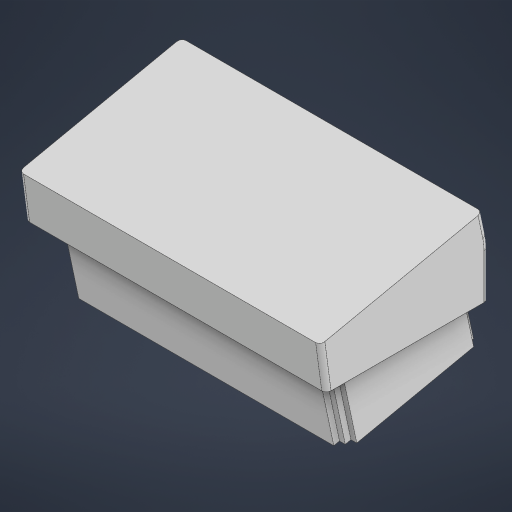
# Autodesk Inventor part: outer
Saved by Autodesk Inventor 2024.2 (Build 282272000, 272)
## iProperties
Created: 2024-08-19
Part Number: outer
Material: Generic
Document SubType Name: Modeling
Designer: Moe
Density: 1 g/cm^3
Appearance: Default
Author: Moe
Autodesk Inventor part; units mm, degrees
ref_plane "YZ Plane" through (0, 0, 0) normal (1, 0, 0) x (0, 1, 0)
ref_plane "XZ Plane" through (0, 0, 0) normal (0, 1, 0) x (-1, 0, 0)
ref_plane "XY Plane" through (0, 0, 0) normal (0, 0, 1) x (1, 0, 0)
sketch "Sketch1" plane through (0, 0, 0) normal (1, 0, 0) x (0, 1, 0)
  line L0 (0, 0) -> (0, -70)
  line L1 (0, 0) -> (70, 0) construction
  line L2 (0, 0) -> (7, 0)
  line L3 (7, 0) -> (21.879, -70)
  line L4 (7, 0) -> (78.5638, 0) construction
  line L5 (21.879, -70) -> (0, -70)
  dimension "d0" = 70
  dimension "d1" = 90
  dimension "d2" = 7
  dimension "d3" = 78
  constraints: 12 end point, 3 horizontal, 2 equal length, 1 point on line, 1 vertical
  measures "d0" distance of L0.start L0.end
  measures "d1" angle of L0 L1
  measures "d2" distance of L0.start L2.end
  measures "d3" angle of L3 L4
extrude "Extrusion1" add sketch "Sketch1" along normal blind 130
sketch "Sketch2" plane through (0, 7, 0) normal (0, 0.9781476, 0.2079117) x (1, 0, 0)
  line L0 (5, 64.9998) -> (125, 64.9998)
  line L1 (125, 64.9998) -> (125, 5)
  line L2 (125, 5) -> (5, 5)
  line L3 (5, 5) -> (5, 64.9998)
  line L4 (0, 71.5638) -> (130, 71.5638) projected
  line L5 (0, 71.5638) -> (0, 0) projected
  line L6 (0, 0) -> (130, 0) projected
  line L7 (130, 71.5638) -> (130, 0) projected
  point P0 (0, -1.4554)
  dimension "d6" = 6.564
  dimension "d7" = 5
  dimension "d8" = 5
  dimension "d9" = 5
  dimension "d71" = 59.9998
  dimension "d72" = 120
  constraints: 8 end point, 2 parallel, 1 horizontal, 1 perpendicular
  measures "d6" distance between parallel lines of L4 L0
  measures "d7" distance between parallel lines of L5 L3
  measures "d8" distance between parallel lines of L6 L2
  measures "d9" distance between parallel lines of L7 L1
  measures "d71" distance of L2.end L0.start
  measures "d72" distance of L1.end L2.end
ref_plane "Work Plane1" through (0, 25, -70) normal (0, -1, 0) x (1, 0, 0)
sketch "Sketch3" plane through (0, 25, -70) normal (0, -1, 0) x (1, 0, 0)
  line L0 (5, 65.1093) -> (5, 6.4206) projected
  line L1 (5, 6.4206) -> (125, 6.4206) projected
  line L2 (125, 65.1093) -> (5, 65.1093) projected
  line L3 (125, 6.4206) -> (125, 65.1093) projected
  line L4 (10, 6.4206) -> (10, 11.4206)
  line L5 (10, 11.4206) -> (5, 11.4206)
  line L6 (5, 65.1093) -> (10, 65.1093)
  line L7 (10, 65.1093) -> (10, 60.1093)
  line L8 (10, 60.1093) -> (5, 60.1093)
  line L9 (5, 60.1093) -> (5, 65.1093)
  line L10 (125, 65.1093) -> (120, 65.1093)
  line L11 (120, 65.1093) -> (120, 60.1093)
  line L12 (120, 60.1093) -> (125, 60.1093)
  line L13 (125, 60.1093) -> (125, 65.1093)
  line L14 (125, 6.4206) -> (120, 6.4206)
  line L15 (120, 6.4206) -> (120, 11.4206)
  line L16 (120, 11.4206) -> (125, 11.4206)
  line L17 (125, 11.4206) -> (125, 6.4206)
  circle A0 centre (7.5, 8.9206) radius 1.1
  circle A1 centre (7.5, 62.6093) radius 1.1
  circle A2 centre (122.5, 62.6093) radius 1.1
  circle A3 centre (122.5, 7.3907) radius 1.1
  point P0 (0, 70)
  dimension "d13" = 5
  dimension "d14" = 5
  dimension "d15" = 5
  dimension "d16" = 5
  dimension "d17" = 5
  dimension "d18" = 5
  dimension "d19" = 5
  dimension "d20" = 5
  dimension "d21" = 2.2
  dimension "d22" = 2.5
  dimension "d23" = 2.5
  dimension "d24" = 2.2
  dimension "d25" = 2.2
  dimension "d26" = 2.2
  constraints: 28 end point, 6 parallel, 5 perpendicular, 4 centre point, 3 horizontal, 2 point on line
  measures "d13" distance of L4.end L5.end
  measures "d14" distance of L4.start L4.end
  measures "d15" distance of L7.end L8.end
  measures "d16" distance of L6.end L7.end
  measures "d17" distance of L12.end L11.end
  measures "d18" distance of L11.end L10.end
  measures "d19" distance of L15.end L16.end
  measures "d20" distance of L14.end L15.end
  measures "d21" diameter of A0
  measures "d22" distance from line of L1 A0.centre
  measures "d23" distance from line of L0 A0.centre
  measures "d24" diameter of A1
  measures "d25" diameter of A2
  measures "d26" diameter of A3
extrude "Extrusion2" cut sketch "Sketch3" along normal blind 22 contours L2 L7 L8 L0 | L8 L7 L2 L11 L12 L3 L16 L15 L1 L4 L5 L0 | L5 L4 L1 L0 | L2 L3 L12 L11 | L15 L16 L3 L1 A3 | A3 L1 | A0 | A1 | A2 picked at (122.1539, 7.5953)
sketch "Sketch4" plane through (0, 7, 0) normal (0, 0.9781476, 0.2079117) x (1, 0, 0)
  line L0 (125, 5) -> (5, 5) projected
  line L1 (5, 5) -> (10, 5)
  line L2 (10, 5) -> (10, 10)
  line L3 (10, 10) -> (5, 10)
  line L4 (5, 10) -> (5, 5)
  line L5 (125, 5) -> (125, 3.9522) projected
  line L6 (125, 5) -> (120, 5)
  line L7 (120, 5) -> (120, 10)
  line L8 (120, 10) -> (125, 10)
  line L9 (125, 10) -> (125, 5)
  line L10 (125, 66.5546) -> (120, 66.5546)
  line L11 (120, 66.5546) -> (120, 61.5546)
  line L12 (120, 61.5546) -> (125, 61.5546)
  line L13 (125, 61.5546) -> (125, 66.5546)
  line L14 (5, 66.5546) -> (10, 66.5546)
  line L15 (10, 66.5546) -> (10, 61.5546)
  line L16 (10, 61.5546) -> (5, 61.5546)
  line L17 (5, 61.5546) -> (5, 66.5546)
  point P0 (0, -1.4554)
  dimension "d27" = 5
  dimension "d28" = 5
  dimension "d29" = 5
  dimension "d30" = 5
  dimension "d31" = 5
  dimension "d32" = 5
  dimension "d33" = 5
  dimension "d34" = 5
  constraints: 32 end point, 8 parallel, 4 horizontal, 4 perpendicular, 1 point on line
  measures "d27" distance of L3.end L2.end
  measures "d28" distance of L2.end L1.end
  measures "d29" distance of L7.end L8.end
  measures "d30" distance of L6.end L7.end
  measures "d31" distance of L12.end L11.end
  measures "d32" distance of L11.end L10.end
  measures "d33" distance of L15.end L16.end
  measures "d34" distance of L14.end L15.end
extrude "Extrusion3" add sketch "Sketch4" against normal blind 8 contours L0 L7 L8 L9 | L0 L4 L3 L2
extrude "Extrusion4" add sketch "Sketch4" against normal blind 20 contours L13 L12 L11 L10 | L14 L15 L16 L17
sketch "Sketch5" plane through (0, 7, 0) normal (0, 0.9781476, 0.2079117) x (1, 0, 0)
  line L0 (5, 10) -> (5, 61.5546) projected
  line L1 (5, 61.5546) -> (10, 61.5546) projected
  line L2 (10, 61.5546) -> (10, 64.9998) projected
  line L3 (10, 64.9998) -> (120, 64.9998) projected
  line L4 (125, 61.5546) -> (125, 10) projected
  line L5 (120, 64.9998) -> (120, 61.5546) projected
  line L6 (120, 61.5546) -> (125, 61.5546) projected
  line L7 (125, 10) -> (120, 10) projected
  line L8 (120, 10) -> (120, 5) projected
  line L9 (125, 5) -> (120, 5) projected
  line L10 (120, 5) -> (10, 5) projected
  line L11 (10, 5) -> (5, 5) projected
  line L12 (10, 5) -> (10, 10) projected
  line L13 (10, 10) -> (5, 10) projected
  line L14 (0, 71.5638) -> (0, 0) projected
  line L15 (0, 0) -> (130, 0) projected
  line L16 (130, 71.5638) -> (130, 0) projected
  line L17 (0, 71.5638) -> (130, 71.5638) projected
  line L18 (7.5, 7.5) -> (122.5, 7.5)
  line L19 (122.5, 7.5) -> (122.5, 64.0546)
  line L20 (122.5, 64.0546) -> (7.5, 64.0546)
  line L21 (7.5, 64.0546) -> (7.5, 7.5)
  point P0 (0, -1.4554)
  point P1 (10, 64.0546)
  point P2 (120, 64.0546)
  point P3 (122.5, 61.5546)
  point P4 (122.5, 10)
  point P5 (7.5, 10)
  point P6 (7.5, 61.5546)
  point P7 (120, 7.5)
  point P8 (10, 7.5)
  constraints: 8 end point, 2 parallel, 1 horizontal, 1 perpendicular
extrude "Extrusion5" add sketch "Sketch5" against normal blind 40 contours L0 L1 L21 L13 | L21 L1 L2 L20 L5 L6 L19 L7 L8 L18 L12 L13 | L21 L20 L2 L1 | L18 L8 L10 L12 | L2 L3 L5 L20 | L8 L7 L19 L18 | L20 L19 L6 L5 | L19 L6 L4 L7
sketch "Sketch6" plane through (125, 0, -11.7113) normal (1, 0, 0) x (0, 0, -1)
  line L0 (-11.7113, 0) -> (76.9148, 0)
  line L1 (76.9148, 0) -> (76.9148, -64.0889)
  line L2 (76.9148, -64.0889) -> (-11.7113, -64.0889)
  line L3 (-11.7113, -64.0889) -> (-11.7113, 0)
  constraints: 8 end point, 2 parallel, 1 horizontal, 1 perpendicular
extrude "Extrusion6" [suppressed]
fillet "Fillet1" [suppressed]
extrude "Extrusion7" add sketch "Sketch2" along normal blind 5.1
extrude "Extrusion8" add sketch "Sketch4" along normal blind 5.1
sketch "Sketch7" plane through (0, 11.9886, 1.0603) normal (0, 0.9781476, 0.2079117) x (1, 0, 0)
  line L0 (130, 0) -> (130, 71.5638) projected
  line L1 (130, 71.5638) -> (0, 71.5638) projected
  line L2 (0, 71.5638) -> (0, 0) projected
  line L3 (0, 0) -> (130, 0) projected
  line L4 (10, 64.9998) -> (120, 64.9998) projected
  line L5 (125, 61.5546) -> (125, 10) projected
  line L6 (120, 64.9998) -> (120, 61.5546) projected
  line L7 (120, 61.5546) -> (125, 61.5546) projected
  line L8 (125, 10) -> (120, 10) projected
  line L9 (120, 10) -> (120, 5) projected
  line L10 (120, 5) -> (10, 5) projected
  line L11 (10, 5) -> (10, 10) projected
  line L12 (10, 10) -> (5, 10) projected
  line L13 (5, 10) -> (5, 61.5546) projected
  line L14 (5, 61.5546) -> (10, 61.5546) projected
  line L15 (10, 61.5546) -> (10, 64.9998) projected
  line L16 (5, 5) -> (5, 3.9522) projected
  line L17 (10, 10) -> (5, 10)
  line L18 (5, 10) -> (5, 5)
  line L19 (5, 5) -> (10, 5)
  line L20 (10, 5) -> (10, 10)
  line L21 (10, 61.5546) -> (5, 61.5546)
  line L22 (5, 61.5546) -> (5, 66.5546)
  line L23 (5, 66.5546) -> (10, 66.5546)
  line L24 (10, 66.5546) -> (10, 61.5546)
  line L25 (120, 61.5546) -> (125, 61.5546)
  line L26 (125, 61.5546) -> (125, 66.5546)
  line L27 (125, 66.5546) -> (120, 66.5546)
  line L28 (120, 66.5546) -> (120, 61.5546)
  line L29 (125, 10) -> (120, 10)
  line L30 (120, 10) -> (120, 5)
  line L31 (120, 5) -> (125, 5)
  line L32 (125, 5) -> (125, 10)
  point P0 (0, -1.4554)
  point P1 (5, 61.5546)
  point P2 (5, 61.5546)
  point P3 (125, 61.5546)
  constraints: 32 end point, 8 parallel, 4 horizontal, 4 perpendicular
extrude "Extrusion9" add sketch "Sketch7" along normal blind 7.5 contours L3 L2 L1 L0 | L4 L6 L7 L5 L8 L9 L10 L11 L12 L13 L14 L15 | L15 L14 L22 L23 L24 | L28 L27 L26 L7 L6 | L12 L11 L19 L18 | L32 L31 L9 L8
fillet "Fillet2" radius 1 4 edges at (120, 22.2922, -59.6793) (120, 11.5734, -9.2513) (10, 11.5734, -9.2513) (10, 22.2922, -59.6793)
fillet "Fillet3" [suppressed]
fillet "Fillet4" [suppressed]
sketch "Sketch8" plane through (130, 0, 0) normal (1, 0, 0) x (0, 0, -1)
  line L0 (-2.6197, 19.3247) -> (0, 0)
  line L1 (0, 7) -> (0, 0) projected
  line L2 (0, 7) -> (-2.6197, 19.3247) projected
  constraints: 2 end point
extrude "Extrusion10" add sketch "Sketch8" against normal blind 130
fillet "Fillet5" radius 25 1 edges at (65, 21.879, -70)
fillet "Fillet6" radius 2 8 edges at (130, 9.6623, 1.3098) (130, 9.6257, -70) (130, 29.3264, -68.417) (130, 21.8646, -69.863) (0, 21.8646, -69.863) (0, 29.3264, -68.417) (0, 9.6257, -70) (0, 9.6623, 1.3098)
sketch "Sketch9" plane through (0, 11.9886, 1.0603) normal (0, 0.9781476, 0.2079117) x (1, 0, 0)
  arc A0 (9, 61.5546) -> (10, 62.5546) centre (9, 62.5546) ccw projected
  line L0 (10, 62.5546) -> (10, 66.5546) projected
  line L1 (10, 66.5546) -> (5, 66.5546) projected
  line L2 (5, 66.5546) -> (5, 61.5546) projected
  line L3 (5, 61.5546) -> (9, 61.5546) projected
  arc A1 (10, 9) -> (9, 10) centre (9, 9) ccw projected
  line L4 (9, 10) -> (5, 10) projected
  line L5 (5, 10) -> (5, 5) projected
  line L6 (5, 5) -> (10, 5) projected
  line L7 (10, 5) -> (10, 9) projected
  arc A2 (121, 10) -> (120, 9) centre (121, 9) ccw projected
  line L8 (120, 9) -> (120, 5) projected
  line L9 (120, 5) -> (125, 5) projected
  line L10 (125, 5) -> (125, 10) projected
  line L11 (125, 10) -> (121, 10) projected
  arc A3 (120, 62.5546) -> (121, 61.5546) centre (121, 62.5546) ccw projected
  line L12 (121, 61.5546) -> (125, 61.5546) projected
  line L13 (125, 61.5546) -> (125, 66.5546) projected
  line L14 (125, 66.5546) -> (120, 66.5546) projected
  line L15 (120, 66.5546) -> (120, 62.5546) projected
  circle A4 centre (7.5, 64.0546) radius 1.1
  circle A5 centre (122.5, 64.0546) radius 1.1
  circle A6 centre (122.5, 7.5) radius 1.1
  circle A7 centre (7.5, 7.5) radius 1.1
  point P0 (0, -1.4554)
  dimension "d57" = 2.2
  dimension "d58" = 2.2
  dimension "d59" = 2.2
  dimension "d60" = 2.2
  constraints: 4 centre point
  measures "d57" diameter of A4
  measures "d58" diameter of A5
  measures "d59" diameter of A6
  measures "d60" diameter of A7
extrude "Extrusion11" cut sketch "Sketch9" against normal blind 10 contours A4 | A5 | A6 | A7
sketch "Sketch10" plane through (10, 3, -65.1093) normal (1, 0, 0) x (0, 0, -1)
  line L0 (0, 5.7706) -> (-2.4544, 17.3177) projected
  line L1 (-2.9435, 17.2137) -> (0, 3.3657) projected
  line L2 (-2.9435, 17.2137) -> (0, 3.3657) projected
  line L3 (-0.009, 17.8375) -> (-2.9435, 17.2137) projected
  line L4 (-0.009, 17.8375) -> (-1.0694, 22.826) projected
  line L5 (-4.982, 21.9944) -> (-1.0694, 22.826) projected
  line L6 (-0.3069, 0) -> (-4.982, 21.9944) projected
  line L7 (0, 0) -> (-0.3069, 0) projected
  line L8 (0, 3.3657) -> (0, 0) projected
  line L9 (0, 5.7706) -> (0, 3.3657) projected
  line L10 (0, 0) -> (-2.4544, 17.3177)
  point P0 (-65.1093, -3)
  constraints: 2 end point
extrude "Extrusion12" [suppressed]
sketch "Sketch11" plane through (128, 19.2514, -70) normal (0, 0, -1) x (-1, 0, 0)
  ellipse E0 centre (117.5, -6.1507) end of major axis (117.5, 1.0663) minor radius 0.5 (118, -6.1507) -> (117.5, 1.0663) ccw projected
  line L0 (118, -16.2514) -> (118, -6.1507) projected
  line L1 (118, -16.2514) -> (8, -16.2514) projected
  line L2 (8, -6.1507) -> (8, -16.2514) projected
  ellipse E1 centre (8.5, -6.1507) end of major axis (8.5, 1.0663) minor radius 0.5 (8.5, 1.0663) -> (8, -6.1507) ccw projected
  line L3 (117.5, 1.0663) -> (8.5, 1.0663) projected
  line L4 (58.25, -12.7514) -> (67.75, -12.7514)
  line L5 (67.75, -12.7514) -> (67.75, -16.2514)
  line L6 (67.75, -16.2514) -> (58.25, -16.2514)
  line L7 (58.25, -16.2514) -> (58.25, -12.7514)
  line L8 (128, -19.2514) -> (128, 0) projected
  point P0 (67.75, -14.5014)
  dimension "d65" = 9.5
  dimension "d66" = 3.5
  dimension "d67" = 0
  dimension "d68" = 60.25
  constraints: 8 end point, 2 parallel, 1 horizontal, 1 midpoint, 1 perpendicular, 2 other
  measures "d65" distance of L5.end L6.end
  measures "d66" distance of L4.end L5.end
  measures "d67" distance between parallel lines of L1 L6
  measures "d68" distance from line of L8 point (67.75, -14.501)
extrude "Extrusion13" cut sketch "Sketch11" against normal blind 9 contours L1 L7 L4 L5
body "Solid1"
